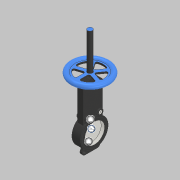
# Autodesk Inventor part: GATE KNIFE VALVE TYPE DN125
Saved by Autodesk Inventor 2017 (Build 210142000, 142)
## iProperties
Created: 2017-11-22
Part Number: GATE KNIFE VALVE TYPE DN125
Material: GG25
Document SubType Name: Modeling
Designer: Demarec
Density: 7.85 g/cm^3
Appearance: Steel - Cast(3)
Description: BELVEN BV50
Catalog Web Link: http://www.pocketbrewery.com
Author: Demarec
Autodesk Inventor part; units mm, degrees
ref_plane "YZ Plane" through (0, 0, 0) normal (1, 0, 0) x (0, 1, 0)
ref_plane "XZ Plane" through (0, 0, 0) normal (0, 1, 0) x (-1, 0, 0)
ref_plane "XY Plane" through (0, 0, 0) normal (0, 0, 1) x (1, 0, 0)
sketch "Sketch1" plane through (0, 0, 0) normal (0, 1, 0) x (-1, 0, 0)
  circle A0 centre (0, 0) radius 80
  circle A1 centre (0, 0) radius 90
  circle A2 centre (0, 0) radius 65
  circle A3 centre (0, 0) radius 105 construction
  line L0 (-16, 63) -> (-16, 570)
  line L1 (-16, 570) -> (0, 570)
  line L2 (0, 570) -> (0, 65)
  line L3 (0, 0) -> (0, 570) construction
  line L4 (0, 46.602497) -> (0, 325.714286)
  circle A4 centre (-40.18176, -97.007351) radius 12
  line L5 (0, 0) -> (-40.18176, -97.007351) construction
  line L6 (-50.375481, -74.580902) -> (-56.811592, -90.119049)
  arc A5 (-56.811592, -90.119049) -> (-40.18176, -115.007351) centre (-40.18176, -97.007351) ccw
  line L7 (-40.18176, -115.007351) -> (0, -115.007351)
  line L8 (0, -115.007351) -> (0, -90)
  line L9 (0, -90) -> (-50.375481, -74.580902)
  circle A6 centre (-110, 325.714286) radius 16
  line L10 (0, 320.380952) -> (-110, 320.380952)
  line L11 (-110, 320.380952) -> (-110, 331.047619)
  line L12 (-110, 331.047619) -> (0, 331.047619)
  line L13 (0, 331.047619) -> (0, 320.380952)
  line L14 (-62.249498, 65) -> (-62.249498, 309.714286)
  line L15 (-62.249498, 309.714286) -> (0, 309.714286)
  line L16 (0, 309.714286) -> (0, 49.053542)
  line L17 (0, 65) -> (-62.249498, 65)
  line L18 (0, 309.714286) -> (0, 65)
  line L19 (0, 0) -> (-40.18176, 97.007351)
  circle A7 centre (-40.18176, 97.007351) radius 12
  arc A8 (-23.022705, 102.444888) -> (-56.159964, 88.718986) centre (-40.18176, 97.007351) ccw
  line L20 (-56.811592, 90.119049) -> (-41.504255, 53.163868)
  line L21 (-41.504255, 53.163868) -> (-8.244592, 66.940471)
  line L22 (-8.244592, 66.940471) -> (-23.551929, 103.895653)
  point P0 (-24.874423, 60.05217)
  dimension "oDiaGasket" = 160
  dimension "oDiaOutside" = 180
  dimension "oDiaInside" = 130
  dimension "oKcircle" = 210
  dimension "oCenterTop" = 570
  dimension "d52" = 32
  dimension "d53" = 10.66667
  dimension "oWheelDia" = 220
  dimension "d58" = 10.66667
  dimension "oHoleDia" = 24
  dimension "d63" = 6
  dimension "oAngleFirstBolt" = 22.5
  dimension "d66" = 325.71429
  dimension "oRibThick" = 16
  dimension "d78" = 22.5
  constraints: 46 end point, 16 point on circle, 9 centre point, 7 parallel, 6 coincident, 6 perpendicular, 4 point on line, 4 tangent, 3 midpoint, 2 collinear, 2 equal radius, 2 horizontal, 1 concentric, 1 vertical
  measures "oDiaGasket" diameter of A0
  measures "oDiaOutside" diameter of A1
  measures "oDiaInside" diameter of A2
  measures "oKcircle" diameter of A3
  measures "oCenterTop" distance from line of L1 L5.start
  measures "d52" diameter of A6
  measures "d53" distance of L10.end L11.end
  measures "oWheelDia" diameter of L11 L3
  measures "d58" distance between parallel lines of L10 L15
  measures "oHoleDia" diameter of A4
  measures "d63" radial gap between concentric circles of A5 A4
  measures "oAngleFirstBolt" angle of L8 L5
  measures "d66" vertical distance of A6.centre L5.start
  measures "oRibThick" distance between parallel lines of L0 L2
  measures "d78" angle of L19 L3
sketch "Sketch2" plane through (0, 0, 0) normal (0, 1, 0) x (-1, 0, 0)
  circle A0 centre (0, 0) radius 90
  circle A1 centre (0, 0) radius 65
  circle A2 centre (0, 0) radius 80
  circle A3 centre (0, 0) radius 90 projected
  circle A4 centre (0, 0) radius 80 projected
  circle A5 centre (0, 0) radius 65 projected
  constraints: 4 coincident, 3 centre point, 3 concentric
extrude "Extrusion4" add sketch "Sketch2" along normal mid plane 56 contours A0 | A2
extrude "Extrusion5" add sketch "Sketch2" along normal mid plane 60 contours A2
sketch "Sketch1 outline for Revolution1" plane through (0, 0, 0) normal (0, 1, 0) x (-1, 0, 0)
  line L0 (-94.915055, 320.380952) -> (-16, 320.380952)
  line L1 (-16, 320.380952) -> (-16, 63)
  arc A0 (-16, 63) -> (0, 65) centre (0, 0) cw
  line L2 (0, 65) -> (0, 570)
  line L3 (0, 570) -> (-16, 570)
  line L4 (-16, 570) -> (-16, 331.047619)
  line L5 (-16, 331.047619) -> (-94.915055, 331.047619)
  arc A1 (-94.915055, 331.047619) -> (-94.915055, 320.380952) centre (-110, 325.714286) ccw
revolve "Revolution1" add sketch "Sketch1 outline for Revolution1" angle 360 about axis through (0, 0, 0) along (0, 0, 1)
extrude "Extrusion8" add sketch "Sketch1" along normal mid plane 15 contours A2 | A1 L8 L7 A5 L6
mirror "Mirror1" about plane through (0, 0, 0) normal (1, 0, 0) of "Extrusion8"
extrude "Extrusion12" add sketch "Sketch1" along normal mid plane 40 contours L2 L17 L21 L22 A0 | A0 L22 L0 A1 L2 | L17 A1 L20 A0 | A0 L20 L17 | L22 L21 L17 L0 A0 | A0 L0 L22 | A1 L0 L15 L2 | L20 A1 L19 A0 | A0 L19 L17 L20 | L14 L15 L0 A1 L22 A8 L20 | L0 L17 L19 A0 | A0 L19 A1 L22 L0 | L22 A1 L0 | L20 A8 L22 A1 | A7
extrude "Extrusion14" add sketch "Sketch1" against normal up to surface (56 mm away) from surface at 28 contours L22 L21 L17 L0 A0 | A0 L0 L22 | L20 A1 L19 A0 | A0 L19 L17 L20 | L17 L19 L21 L20 | L0 L17 L19 A0 | A0 L19 A1 L22 L0 | L21 L0 L17 | L20 A8 L22 A1 | L17 L0 L21 L19
mirror "Mirror2" about plane through (0, 0, 65) normal (-1, 0, 0) of "Extrusion12", "Extrusion14"
chamfer "Chamfer2" distance 40 angle 45 2 edges at (-62.2495, 0, 309.7143) (62.2495, 0, 309.7143)
sketch "Sketch5" plane through (0, 0, 331.047619) normal (0, 0, 1) x (1, 0, 0)
  line L0 (30.122147, 8.09017) -> (64.699456, 33.212055)
  arc A0 (79.998286, 28.475268) -> (64.699456, 33.212055) centre (70.577308, 25.121885) ccw
  arc A1 (30.122147, 8.09017) -> (30.122147, -8.09017) centre (36, 0) ccw
  line L1 (30.122147, -8.09017) -> (64.699456, -33.212055)
  arc A2 (64.699456, -33.212055) -> (79.998286, -28.475268) centre (70.577308, -25.121885) ccw
  arc A3 (79.998286, -28.475268) -> (79.998286, 28.475268) centre (0, 0) ccw
  line L2 (0, 0) -> (36, 0)
  circle A4 centre (0, 0) radius 94.915055
  circle A5 centre (0, 0) radius 84.915055
  circle A6 centre (0, 0) radius 16
  circle A7 centre (0, 0) radius 26
  dimension "d68" = 72
  dimension "d69" = 36
  dimension "d70" = 10
  dimension "d71" = 10
  dimension "d72" = 10
  constraints: 8 point on circle, 7 tangent, 6 centre point, 6 end point, 2 equal radius, 1 coincident, 1 concentric, 1 equal length, 1 horizontal
  measures "d68" angle of L1 L0
  measures "d69" angle of L2 L0
  measures "d70" radial gap between concentric circles of A4 A5
  measures "d71" radial gap between concentric circles of A6 A7
  measures "d72" radius of A1
sketch "Sketch5 outline for Extrusion13" plane through (0, 0, 331.047619) normal (0, 0, 1) x (1, 0, 0)
  line L0 (30.122147, 8.09017) -> (64.699456, 33.212055)
  arc A0 (64.699456, 33.212055) -> (79.998286, 28.475268) centre (70.577308, 25.121885) cw
  arc A1 (79.998286, 28.475268) -> (79.998286, -28.475268) centre (0, 0) cw
  arc A2 (79.998286, -28.475268) -> (64.699456, -33.212055) centre (70.577308, -25.121885) cw
  line L1 (64.699456, -33.212055) -> (30.122147, -8.09017)
  arc A3 (30.122147, -8.09017) -> (30.122147, 8.09017) centre (36, 0) cw
extrude "Extrusion13" cut sketch "Sketch5 outline for Extrusion13" against normal blind 20
pattern_circular "Circular Pattern2" count 5 over 360 about axis through (0, 0, 316.5) along (0, 0, 1) of "Extrusion13"
body "Solid2"
